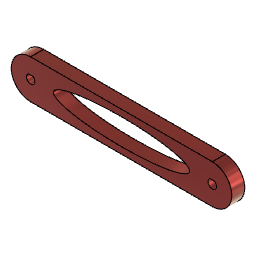
haste-conectora (Autodesk Fusion 360 design; units mm, degrees)
Autodesk Fusion 360 part; units mm, degrees
note: some values were not read from the file. Set by a fixed rule: which sketch regions a step uses.
sketch "Sketch2" plane through (0, 0, 0) normal (0, 1, 0) x (1, 0, 0)
  line L0 (0, -50) -> (80, -50)
  line L1 (0, -50) -> (-80, -50)
  line L2 (-80, -52.8) -> (80, -52.8)
  circle A0 centre (70, -50) radius 3.3
  circle A1 centre (-70, -50) radius 3.25
  line L3 (-70, -65) -> (70, -65)
  arc A2 (70, -65) -> (70, -35) centre (70, -50) ccw
  line L4 (70, -35) -> (-70, -35)
  arc A3 (-70, -35) -> (-70, -65) centre (-70, -50) ccw
  line L5 (-70, -50) -> (70, -50) construction
  ellipse E0 centre (0, -50) end of major axis (52.5047, -50) minor radius 10
  line L6 (-52.5047, -50) -> (52.5047, -50)
  line L7 (0, -60) -> (0, -40)
  circle A4 centre (-70, -50) radius 0.75
  circle A5 centre (70, -50) radius 0.75
  dimension "d7" = 80
  dimension "d8" = 80
  dimension "d9" = 2.8
  dimension "d10" = 6.6
  dimension "d11" = 6.5
  dimension "d12" = 30
  dimension "d13" = 20
  dimension "d14" = 1.5
  dimension "d15" = 1.5
  constraint horizontal L0
  constraint parallel L0 L1
  constraint horizontal L2
  constraint coincident L0 A0.centre
  constraint coincident L1 A1.centre
  constraint tangent L3 A2
  constraint tangent A2 L4
  constraint parallel L3 L4
  constraint tangent L4 A3
  constraint tangent L3 A3
  constraint coincident A0.centre A2.centre
  constraint parallel L0 L5
  constraint coincident A1.centre A3.centre
  constraint coincident E0 L6.start
  constraint coincident E0 L6.end
  constraint coincident E0 L7.start
  constraint coincident E0 L7.end
  constraint coincident L0.start L1.start
  constraint parallel L5 L6
  constraint concentric A1 A4
  constraint concentric A2 A5
  measures "d7" distance of L0.start L0.end
  measures "d8" distance of L0.start L1.end
  measures "d9" distance of L0 L2
  measures "d10" diameter of A0
  measures "d11" diameter of A1
  measures "d12" diameter of A2
  measures "d14" diameter of A4
  measures "d15" diameter of A5
extrude "Extrude1" add sketch "Sketch2" along normal blind 10 contours L0 L2 A0 E0 | L1 L2 A1 E0 | L0 A0 A5 | L0 L2 A0 A5 | L1 L2 A1 A4 | L1 A1 A4 | L0 A5 | L0 A5 | L2 A0 | L1 A4 | L1 A4 | L2 A1 | L3 A2 L4 A3
extrude "Extrude2" cut sketch "Sketch2" along normal blind 7 contours L0 A0 A5 | L0 L2 A0 A5 | L1 L2 A1 A4 | L1 A1 A4
extrude "Extrude3" cut sketch "Sketch2" along normal blind 3 contours L0 A5 | L0 A5 | L1 A4 | L1 A4
